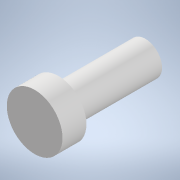
# Autodesk Inventor part: bolt
Saved by Autodesk Inventor 2021 (Build 250183000, 183)
## iProperties
Created: 2021-07-16
Part Number: bolt
Material: Generic
Document SubType Name: Modeling
Designer: Dell
Density: 1 g/cm^3
Appearance: Default
Author: Dell
Autodesk Inventor part; units mm, degrees
ref_plane "YZ Plane" through (0, 0, 0) normal (1, 0, 0) x (0, 1, 0)
ref_plane "XZ Plane" through (0, 0, 0) normal (0, 1, 0) x (-1, 0, 0)
ref_plane "XY Plane" through (0, 0, 0) normal (0, 0, 1) x (1, 0, 0)
sketch "Sketch1" plane through (0, 0, 0) normal (0, 0, 1) x (1, 0, 0)
  circle A0 centre (16.3737, -3.1223) radius 0.489
  point P0 (0, 0)
  constraints: 1 centre point
extrude "Extrusion1" add sketch "Sketch1" against normal blind 2.54
sketch "Sketch2" plane through (16.3737, -3.1223, 0) normal (0, 0, 1) x (1, 0, 0)
  circle A0 centre (0, 0) radius 0.8152
  point P0 (-16.3737, 3.1223)
  constraints: 1 centre point
extrude "Extrusion2" add sketch "Sketch2" along normal blind 0.7
body "Solid1"
